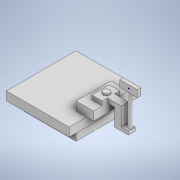
# Autodesk Inventor part: upper plate
Saved by Autodesk Inventor 2021 (Build 250183000, 183)
## iProperties
Created: 2021-06-22
Part Number: upper plate
Material: Generic
Document SubType Name: Modeling
Designer: Rajeev
Density: 1 g/cm^3
Appearance: Default
Author: Rajeev
Autodesk Inventor part; units mm, degrees
ref_plane "YZ Plane" through (0, 0, 0) normal (1, 0, 0) x (0, 1, 0)
ref_plane "XZ Plane" through (0, 0, 0) normal (0, 1, 0) x (-1, 0, 0)
ref_plane "XY Plane" through (0, 0, 0) normal (0, 0, 1) x (1, 0, 0)
sketch "Sketch1" plane through (0, 0, 0) normal (0, 1, 0) x (-1, 0, 0)
  line L0 (30.8368, 11.4286) -> (-9.1632, 11.4286)
  line L1 (-9.1632, 11.4286) -> (-9.1632, -28.5714)
  line L2 (-9.1632, -28.5714) -> (30.8368, -28.5714)
  line L3 (30.8368, -28.5714) -> (30.8368, 11.4286)
  point P0 (0, 0)
  dimension "d0" = 40
  dimension "d1" = 40
  constraints: 8 end point, 2 parallel, 1 horizontal, 1 perpendicular
  measures "d0" distance of L2.end L1.end
  measures "d1" distance of L1.end L0.end
extrude "Extrusion1" add sketch "Sketch1" along normal blind 5
sketch "Sketch7" plane through (9.1632, 0, -28.5714) normal (1, 0, 0) x (0, 0, -1)
  point P0 (-28.5714, 0)
sketch "Sketch8" plane through (0, 0, 0) normal (0, -1, 0) x (1, 0, 0)
  point P0 (0, 0)
sketch "Sketch11" plane through (0, 5, 0) normal (0, 1, 0) x (1, 0, 0)
  line L0 (9.1632, -11.4286) -> (9.1632, 28.5714) projected
  line L1 (9.1632, 18.5714) -> (-0.8368, 18.5714)
  line L2 (-0.8368, 18.5714) -> (-0.8368, -1.4286)
  line L3 (-0.8368, -1.4286) -> (9.1632, -1.4286)
  line L4 (9.1632, -1.4286) -> (9.1632, 18.5714)
  line L5 (-30.8368, -11.4286) -> (9.1632, -11.4286) projected
  point P0 (0, 0)
  dimension "d29" = 10
  dimension "d30" = 20
  dimension "d31" = 10
  constraints: 8 end point, 2 parallel, 1 horizontal, 1 perpendicular, 1 point on line
  measures "d29" distance of L1.start L1.end
  measures "d30" distance of L1.end L2.end
  measures "d31" distance between parallel lines of L5 L3
extrude "Extrusion7" add sketch "Sketch11" along normal blind 5
sketch "Sketch12" plane through (0, 10, 0) normal (0, 1, 0) x (1, 0, 0)
  line L0 (9.1632, -1.4286) -> (9.1632, 18.5714) projected
  line L1 (3.175, 13.5714) -> (9.1632, 13.5714)
  line L2 (9.1632, 13.5714) -> (9.1632, 3.5714)
  line L3 (9.1632, 3.5714) -> (3.175, 3.5714)
  line L4 (3.175, 3.5714) -> (3.175, 13.5714)
  line L5 (9.1632, 18.5714) -> (-0.8368, 18.5714) projected
  point P0 (0, 0)
  dimension "d34" = 10
  dimension "d35" = 5
  constraints: 8 end point, 2 parallel, 1 horizontal, 1 perpendicular, 1 point on line
  measures "d34" distance of L3.end L1.start
  measures "d35" distance between parallel lines of L1 L5
extrude "Extrusion8" add sketch "Sketch12" along normal blind 2.5
sketch "Sketch13" plane through (9.1632, 0, 11.4286) normal (1, 0, 0) x (0, 0, -1)
  line L0 (25, 12.5) -> (15, 12.5) projected
  line L1 (30, 10) -> (10, 10) projected
  line L2 (18, 12.5) -> (22, 12.5)
  line L3 (22, 12.5) -> (22, 10)
  line L4 (22, 10) -> (18, 10)
  line L5 (18, 10) -> (18, 12.5)
  line L6 (15, 10) -> (15, 12.5) projected
  point P0 (11.4286, 0)
  dimension "d38" = 4
  dimension "d39" = 3
  constraints: 8 end point, 2 parallel, 2 point on line, 1 horizontal, 1 perpendicular
  measures "d38" distance of L2.end L2.start
  measures "d39" distance between parallel lines of L6 L5
extrude "Extrusion9" add sketch "Sketch13" along normal blind 4 contours L3 L1 L5 L0
sketch "Sketch14" plane through (0, 0, 0) normal (0, -1, 0) x (1, 0, 0)
  line L0 (4.1632, 6.4286) -> (-25.8368, 6.4286)
  line L1 (-25.8368, 6.4286) -> (-25.8368, -23.5714)
  line L2 (-25.8368, -23.5714) -> (4.1632, -23.5714)
  line L3 (4.1632, -23.5714) -> (4.1632, 6.4286)
  line L4 (9.1632, 11.4286) -> (9.1632, -28.5714) projected
  line L5 (9.1632, -28.5714) -> (-30.8368, -28.5714) projected
  point P0 (0, 0)
  dimension "d42" = 30
  dimension "d43" = 30
  dimension "d44" = 5
  dimension "d45" = 5
  constraints: 8 end point, 2 parallel, 1 horizontal, 1 perpendicular
  measures "d42" distance of L2.end L0.start
  measures "d43" distance of L0.start L0.end
  measures "d44" distance between parallel lines of L3 L4
  measures "d45" distance between parallel lines of L2 L5
extrude "Extrusion10" add sketch "Sketch14" along normal blind 4
sketch "Sketch15" plane through (13.1632, 0, 11.4286) normal (1, 0, 0) x (0, 0, -1)
  line L0 (25, 12.5) -> (15, 12.5) projected
  line L1 (18.0261, 12.5) -> (22.0261, 12.5)
  line L2 (22.0261, 12.5) -> (22.0261, -15.875)
  line L3 (22.0261, -15.875) -> (18.0261, -15.875)
  line L4 (18.0261, -15.875) -> (18.0261, 12.5)
  point P0 (11.4286, 0)
  dimension "d48" = 4
  constraints: 8 end point, 2 parallel, 1 horizontal, 1 perpendicular, 1 point on line
  measures "d48" distance of L2.end L3.end
extrude "Extrusion11" add sketch "Sketch15" along normal blind 4
sketch "Sketch30" plane through (13.1632, -15.875, -6.5975) normal (0, 0, 1) x (1, 0, 0)
  point P0 (-13.1632, 15.875)
sketch "Sketch31" plane through (17.1632, 0, 11.4286) normal (1, 0, 0) x (0, 0, -1)
  line L0 (18.0261, 10) -> (18.0261, -15.875) projected
  line L1 (22.0261, -15.875) -> (22.0261, 12.5) projected
  line L2 (18.0261, -15.875) -> (22.0261, -15.875)
  line L3 (22.0261, -15.875) -> (22.0261, -13.875)
  line L4 (22.0261, -13.875) -> (18.0261, -13.875)
  line L5 (18.0261, -13.875) -> (18.0261, -15.875)
  line L6 (18.0261, 12.5) -> (22.0261, 12.5)
  line L7 (22.0261, 12.5) -> (22.0261, -15.875)
  line L8 (22.0261, -15.875) -> (18.0261, -15.875)
  line L9 (18.0261, -15.875) -> (18.0261, 12.5)
  point P0 (11.4286, 0)
  dimension "d75" = 2
  constraints: 16 end point, 4 parallel, 2 horizontal, 2 perpendicular, 1 point on line
  measures "d75" distance of L1.start L3.end
extrude "Extrusion21" cut sketch "Sketch31" against normal blind 4 contours L9 L6 L1 L4 L0
sketch "Sketch32" plane through (17.1632, 0, 11.4286) normal (1, 0, 0) x (0, 0, -1)
  line L0 (15.875, -11.1125) -> (23.8125, -11.1125)
  line L1 (23.8125, -11.1125) -> (23.8125, -20.6375)
  line L2 (23.8125, -20.6375) -> (15.875, -20.6375)
  line L3 (15.875, -20.6375) -> (15.875, -11.1125)
  point P0 (11.4286, 0)
  constraints: 8 end point, 2 parallel, 1 horizontal, 1 perpendicular
extrude "Extrusion22" cut sketch "Sketch32" against normal blind 4
sketch "Sketch33" plane through (13.1632, 0, 11.4286) normal (1, 0, 0) x (0, 0, -1)
  line L0 (25, 12.5) -> (15, 12.5) projected
  line L1 (5, 0) -> (35, 0) projected
  line L2 (18, 12.5) -> (22, 12.5)
  line L3 (22, 12.5) -> (22, 0)
  line L4 (22, 0) -> (18, 0)
  line L5 (18, 0) -> (18, 12.5)
  line L6 (18, 12.5) -> (18, 10) projected
  point P0 (11.4286, 0)
  dimension "d80" = 4
  dimension "d81" = 0
  constraints: 8 end point, 2 parallel, 2 point on line, 1 horizontal, 1 perpendicular
  measures "d80" distance of L3.end L4.end
  measures "d81" distance between parallel lines of L5 L6
extrude "Extrusion23" add sketch "Sketch33" along normal blind 4
sketch "Sketch34" plane through (17.1632, 0, 11.4286) normal (1, 0, 0) x (0, 0, -1)
  line L0 (5, 0) -> (35, 0) projected
  line L1 (22, 0) -> (22, 10) projected
  line L2 (18, 0) -> (22, 0)
  line L3 (22, 0) -> (22, 2)
  line L4 (22, 2) -> (18, 2)
  line L5 (18, 2) -> (18, 0)
  line L6 (18, 12.5) -> (18, 0) projected
  point P0 (11.4286, 0)
  dimension "d84" = 2
  dimension "d85" = 0
  constraints: 8 end point, 2 parallel, 2 point on line, 1 horizontal, 1 perpendicular
  measures "d84" distance of L1.start L3.end
  measures "d85" distance between parallel lines of L6 L5
extrude "Extrusion24" add sketch "Sketch34" along normal blind 2
sketch "Sketch35" plane through (17.1632, 2, -6.5714) normal (0, 1, 0) x (1, 0, 0)
  point P0 (-17.1632, -6.5714)
sketch "Sketch36" plane through (19.1632, 0, 11.4286) normal (1, 0, 0) x (0, 0, -1)
  line L0 (22, 0) -> (22, 10) projected
  line L1 (22, 2) -> (18, 2)
  line L2 (18, 2) -> (18, 0)
  line L3 (18, 0) -> (22, 0)
  line L4 (22, 0) -> (22, 2)
  point P0 (11.4286, 0)
  dimension "d88" = 4
  dimension "d89" = 2
  constraints: 8 end point, 2 parallel, 1 horizontal, 1 perpendicular, 1 point on line
  measures "d88" distance of L2.end L3.end
  measures "d89" distance of L1.end L2.end
extrude "Extrusion25" add sketch "Sketch36" along normal blind 2
sketch "Sketch37" plane through (17.1632, 2, -6.5714) normal (0, 1, 0) x (1, 0, 0)
  line L0 (2, 3.175) -> (4, 3.175)
  line L1 (4, 3.175) -> (4, 1.175)
  line L2 (4, 1.175) -> (2, 1.175)
  line L3 (2, 1.175) -> (2, 3.175)
  line L4 (4, 4) -> (4, 0) projected
  point P0 (-17.1632, -6.5714)
  dimension "d92" = 2
  dimension "d93" = 2
  dimension "d94" = 0
  constraints: 8 end point, 2 parallel, 1 horizontal, 1 perpendicular
  measures "d92" distance of L0.end L1.end
  measures "d93" distance of L1.end L2.end
  measures "d94" distance between parallel lines of L1 L4
extrude "Extrusion26" add sketch "Sketch37" along normal blind 18
sketch "Sketch38" plane through (17.1632, 20, -6.5714) normal (0, 1, 0) x (1, 0, 0)
  line L0 (-2, 3.175) -> (8, 3.175)
  line L1 (8, 3.175) -> (8, 1.175)
  line L2 (8, 1.175) -> (-2, 1.175)
  line L3 (-2, 1.175) -> (-2, 3.175)
  line L4 (4, 3.175) -> (2, 3.175) projected
  line L5 (4, 1.175) -> (4, 3.175) projected
  line L6 (2, 3.175) -> (2, 1.175) projected
  point P0 (-17.1632, -6.5714)
  dimension "d97" = 2
  dimension "d98" = 0
  dimension "d99" = 4
  dimension "d100" = 4
  constraints: 8 end point, 2 parallel, 1 horizontal, 1 perpendicular
  measures "d97" distance of L1.end L0.end
  measures "d98" distance between parallel lines of L4 L0
  measures "d99" distance between parallel lines of L1 L5
  measures "d100" distance between parallel lines of L3 L6
extrude "Extrusion27" add sketch "Sketch38" along normal blind 4
fillet "Fillet1" radius 1 4 edges at (21.1632, 11, -9.7464) (19.1632, 11, -9.7464) (19.1632, 11, -7.7464) (21.1632, 11, -7.7464)
sketch "Sketch40" plane through (15.1632, 24, -7.7464) normal (0, 0, 1) x (1, 0, 0)
  circle A0 centre (5.0665, -1.7928) radius 0.3
  point P0 (-15.1632, -24)
  dimension "d110" = 0.6
  constraints: 1 centre point
  measures "d110" diameter of A0
extrude "Extrusion29" cut sketch "Sketch40" against normal blind 100
sketch "Sketch41" plane through (15.1632, 24, -7.7464) normal (0, 0, 1) x (1, 0, 0)
  circle A0 centre (5.0665, -1.7928) radius 0.3 projected
  circle A1 centre (5.0665, -1.7928) radius 0.3
  point P0 (-15.1632, -24)
  constraints: 1 centre point, 1 coincident
sketch "Sketch42" plane through (0, -4, 0) normal (0, -1, 0) x (1, 0, 0)
  line L0 (4.1632, 6.4286) -> (4.1632, -23.5714) projected
  line L1 (-25.8368, 6.4286) -> (4.1632, 6.4286) projected
  line L2 (4.1632, -23.5714) -> (-25.8368, -23.5714)
  line L3 (-25.8368, -23.5714) -> (-25.8368, 6.4286)
  line L4 (-25.8368, 6.4286) -> (4.1632, 6.4286)
  line L5 (4.1632, 6.4286) -> (4.1632, -23.5714)
  point P0 (0, 0)
  constraints: 8 end point, 2 parallel, 1 horizontal, 1 perpendicular
extrude "Extrusion30" add sketch "Sketch42" along normal blind 10
sketch "Sketch43" plane through (0, 12.5, 0) normal (0, 1, 0) x (1, 0, 0)
  line L0 (4.973, 9.5849) -> (6.6857, 10.5243)
  line L1 (6.6857, 10.5243) -> (8.3555, 9.5108)
  line L2 (8.3555, 9.5108) -> (8.3127, 7.5579)
  line L3 (8.3127, 7.5579) -> (6.6, 6.6185)
  line L4 (6.6, 6.6185) -> (4.9302, 7.632)
  line L5 (4.9302, 7.632) -> (4.973, 9.5849)
  point P0 (0, 0)
  point P1 (6.6429, 8.5714)
  constraints: 12 end point, 13 other
extrude "Extrusion31" add sketch "Sketch43" along normal blind 1
sketch "Sketch44" plane through (0, 0, 0) normal (0, -1, 0) x (1, 0, 0)
  circle A0 centre (6.6857, -8.642) radius 1.5
  point P0 (0, 0)
  dimension "d117" = 3
  constraints: 1 centre point
  measures "d117" diameter of A0
extrude "Extrusion32" add sketch "Sketch44" along normal blind 1
sketch "Sketch45" plane through (4.1632, 0, -23.5714) normal (0, 0, -1) x (-1, 0, 0)
  line L0 (30, -14) -> (0, -14) projected
  line L1 (30, 0) -> (30, -14) projected
  line L2 (0, -14) -> (30, -14)
  line L3 (30, -14) -> (30, -5.1197)
  line L4 (30, -5.1197) -> (0, -5.1197)
  line L5 (0, -5.1197) -> (0, -14)
  point P0 (4.1632, 0)
  constraints: 8 end point, 2 parallel, 1 horizontal, 1 perpendicular, 1 point on line
extrude "Extrusion33" cut sketch "Sketch45" against normal blind 100
sketch "Sketch46" plane through (-25.8368, -5.1197, -23.5714) normal (0, -1, 0) x (1, 0, 0)
  point P0 (25.8368, 23.5714)
sketch "Sketch47" plane through (9.1632, 0, 11.4286) normal (1, 0, 0) x (0, 0, -1)
  line L0 (35, -5.1197) -> (5, -5.1197) projected
  line L1 (40, 5) -> (0, 5) projected
  line L2 (35, -5.1197) -> (0, -5.1197)
  line L3 (0, -5.1197) -> (0, 5)
  line L4 (0, 5) -> (35, 5)
  line L5 (30, 5) -> (40, 5) projected
  line L6 (35, 5) -> (40, 5)
  line L7 (40, 0) -> (40, 5) projected
  line L8 (40, 5) -> (40, -5.1197)
  line L9 (40, -5.1197) -> (33.3375, -5.1197)
  point P0 (11.4286, 0)
  point P1 (5, -5.1197)
  constraints: 12 end point, 1 horizontal, 1 parallel, 1 perpendicular, 1 point on line, 1 vertical
extrude "Extrusion34" cut sketch "Sketch47" against normal blind 4
body "Solid1"
